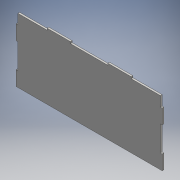
# Autodesk Inventor part: InSupp
Saved by Autodesk Inventor 2016 (Build 200138000, 138)
## iProperties
Created: 2016-12-13
Part Number: InSupp
Material: Generic
Document SubType Name: Modeling
Designer: NacostaMobile
Density: 1 g/cm^3
Appearance: Default
Author: NacostaMobile
Autodesk Inventor part; units mm, degrees
ref_plane "YZ Plane" through (0, 0, 0) normal (1, 0, 0) x (0, 1, 0)
ref_plane "XZ Plane" through (0, 0, 0) normal (0, 1, 0) x (-1, 0, 0)
ref_plane "XY Plane" through (0, 0, 0) normal (0, 0, 1) x (1, 0, 0)
sketch "Sketch1" plane through (0, 0, 0) normal (0, 1, 0) x (-1, 0, 0)
  line L0 (-247, -113) -> (-3, -113)
  line L1 (-3, -113) -> (0, -113)
  line L2 (0, -113) -> (0, -88)
  line L3 (0, -88) -> (-3, -88)
  line L4 (-3, -88) -> (-3, -45)
  line L5 (-3, -45) -> (0, -45)
  line L6 (0, -45) -> (0, -20)
  line L7 (0, -20) -> (-3, -20)
  line L8 (-247, -113) -> (-250, -113)
  line L9 (-250, -113) -> (-250, -88)
  line L10 (-250, -88) -> (-247, -88)
  line L11 (-247, -88) -> (-247, -45)
  line L12 (-247, -88) -> (-204, -88) construction
  line L13 (-247, -45) -> (-250, -45)
  line L14 (-250, -45) -> (-250, -20)
  line L15 (-250, -20) -> (-247, -20)
  line L16 (-3, -88) -> (-3, -45)
  line L17 (-3, -20) -> (-3, -3)
  line L18 (-247, -3) -> (-247, -20)
  line L19 (-247, -45) -> (-247, -88)
  line L20 (-3, -3) -> (-53, -3)
  line L21 (-53, -3) -> (-53, 0)
  line L22 (-53, 0) -> (-93, 0)
  line L23 (-93, 0) -> (-93, -3)
  line L24 (-247, -3) -> (-197, -3)
  line L25 (-197, -3) -> (-197, 0)
  line L26 (-197, 0) -> (-157, 0)
  line L27 (-157, 0) -> (-157, -3)
  line L28 (-197, -3) -> (-247, -3)
  line L29 (-3, -3) -> (-53, -3)
  line L30 (-93, -3) -> (-157, -3)
  point P0 (0, 0)
  dimension "d3" = 244
  dimension "d4" = 110
  dimension "d5" = 244
  dimension "d6" = 3
  dimension "d7" = 25
  dimension "d8" = 90
  dimension "d9" = 3
  dimension "d10" = 43
  dimension "d12" = 25
  dimension "d13" = 3
  dimension "d14" = 25
  dimension "d15" = 3
  dimension "d16" = 43
  dimension "d17" = 90
  dimension "d18" = 3
  dimension "d19" = 25
  dimension "d22" = 50
  dimension "d23" = 3
  dimension "d24" = 40
  dimension "d25" = 50
  dimension "d26" = 3
  dimension "d27" = 40
  constraints: 62 end point, 19 perpendicular, 5 parallel, 3 point on line, 2 collinear, 2 horizontal, 2 vertical
  measures "d3" distance of L17.end L18.start
  measures "d4" distance of L18.start L0.start
  measures "d5" distance of L0.start L0.end
  measures "d6" distance of L0.end L1.end
  measures "d7" distance of L1.end L2.end
  measures "d8" angle of L2 L1
  measures "d9" distance of L3.end L2.end
  measures "d10" distance of L3.end L4.end
  measures "d12" distance of L5.end L6.end
  measures "d13" distance of L0.start L8.end
  measures "d14" distance of L8.end L9.end
  measures "d15" distance of L10.end L9.end
  measures "d16" distance of L10.end L11.end
  measures "d17" angle of L12 L11
  measures "d18" distance of L11.end L13.end
  measures "d19" distance of L13.end L14.end
  measures "d22" distance of L17.end L20.end
  measures "d23" distance of L20.end L21.end
  measures "d24" distance of L21.end L22.end
  measures "d25" distance of L18.start L24.end
  measures "d26" distance of L24.end L25.end
  measures "d27" distance of L25.end L26.end
extrude "Extrusion1" add sketch "Sketch1" along normal blind 3
body "Solid1"
